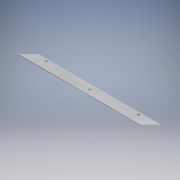
# Autodesk Inventor part: side plate
Saved by Autodesk Inventor 2016 (Build 200138000, 138)
## iProperties
Created: 2016-01-16
Part Number: side plate
Material: Aluminum 6061
Document SubType Name: Modeling
Designer: gus
Density: 2.7 g/cm^3
Appearance: Aluminum - Flat
Mass: 328.58 g
Surface Area: 822.004 cm^2
Volume: 121.696 cm^3
Author: gus
Autodesk Inventor part; units mm, degrees
ref_plane "YZ Plane" through (0, 0, 0) normal (1, 0, 0) x (0, 1, 0)
ref_plane "XZ Plane" through (0, 0, 0) normal (0, 1, 0) x (-1, 0, 0)
ref_plane "XY Plane" through (0, 0, 0) normal (0, 0, 1) x (1, 0, 0)
sketch "Sketch1" plane through (0, 0, 0) normal (0, 1, 0) x (-1, 0, 0)
  line L0 (0, 0) -> (762, 0)
  line L1 (762, 0) -> (762, 50.8)
  line L2 (762, 50.8) -> (0, 50.8)
  line L3 (0, 50.8) -> (0, 0)
  dimension "d0" = 762
  dimension "d1" = 50.8
  constraints: 8 end point, 2 parallel, 1 horizontal, 1 perpendicular
  measures "d0" distance of L2.end L1.end
  measures "d1" distance of L1.end L0.end
extrude "Extrusion1" add sketch "Sketch1" along normal blind 3.175
sketch "Sketch2" plane through (0, 3.175, 0) normal (0, 1, 0) x (1, 0, 0)
  circle A0 centre (-381, -25.4) radius 6.35
  line L0 (0, 0) -> (-762, 0) projected
  line L1 (0, -50.8) -> (0, 0) projected
  circle A1 centre (-152.7531, -12.7) radius 6.35
  line L2 (-762, -50.8) -> (0, -50.8) projected
  circle A2 centre (-609.2469, -12.7) radius 6.35
  dimension "d4" = 12.7
  dimension "d5" = 25.4
  dimension "d6" = 381
  dimension "d9" = 12.7
  dimension "d10" = 38.1
  dimension "d11" = 228.6
  dimension "d12" = 12.7
  dimension "d13" = 38.1
  dimension "d14" = 228.6
  constraints: 3 centre point
  measures "d4" diameter of A0
  measures "d5" distance from line of L0 A0.centre
  measures "d6" distance from line of A0.centre L1
  measures "d9" diameter of A1
  measures "d10" distance from line of L2 A1.centre
  measures "d11" distance of A0.centre A1.centre
  measures "d12" diameter of A2
  measures "d13" distance from line of L2 A2.centre
  measures "d14" distance of A0.centre A2.centre
extrude "Extrusion2" cut sketch "Sketch2" against normal blind 3.175
body "Solid1"
